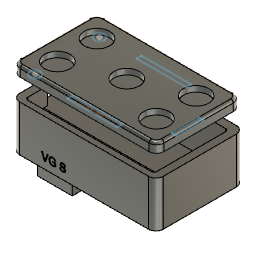
ESPBox and Lid (Autodesk Fusion 360 design; units mm, degrees)
Autodesk Fusion 360 part; units mm, degrees
sketch "Skizze1" plane through (0, 0, 0) normal (0, 0, 1) x (1, 0, 0) in component "Box1"
  line L0 (29, 17.25) -> (-29, 17.25)
  line L1 (-29, 17.25) -> (-29, -17.25)
  line L2 (-29, -17.25) -> (29, -17.25)
  line L3 (29, -17.25) -> (29, 17.25)
  line L4 (29, 17.25) -> (-29, -17.25) construction
  line L5 (-29, 17.25) -> (29, -17.25) construction
  dimension "d1" = 58
  dimension "d2" = 34.5
  constraint horizontal L0
  constraint perpendicular L0 L1
  constraint parallel L0 L2
  constraint parallel L1 L3
  constraint coincident L4 origin
  constraint coincident L5 origin
  measures "d1" distance of L1.end L2.end
  measures "d2" distance of L0.end L1.end
extrude "Extrusion1" add sketch "Skizze1" along normal blind 18.5 makes body 1 in component "Box1"
sketch "Skizze2" plane through (0, 0, 18.5) normal (0, 0, 1) x (-1, 0, 0) in component "Box1"
  line L0 (-29, 17.25) -> (-29, -17.25)
  line L1 (-29, -17.25) -> (29, -17.25)
  line L2 (29, -17.25) -> (29, 17.25)
  line L3 (29, 17.25) -> (-29, 17.25)
  line L4 (-26, -15) -> (26, -15)
  line L5 (26, -15) -> (26, 15)
  line L6 (26, 15) -> (-26, 15)
  line L7 (-26, 15) -> (-26, -15)
  line L8 (-26, -15) -> (26, 15) construction
  line L9 (26, -15) -> (-26, 15) construction
  dimension "d5" = 52
  dimension "d6" = 30
  constraint horizontal L4
  constraint perpendicular L4 L5
  constraint parallel L4 L6
  constraint parallel L5 L7
  constraint coincident L8 origin
  constraint coincident L9 origin
  measures "d5" distance of L5.end L6.end
  measures "d6" distance of L4.end L5.end
extrude "Extrusion2" cut sketch "Skizze2" against normal up to surface (15.5 mm away) contours L4 L5 L6 L7 bodies 1 in component "Box1"
fillet "Abrundung1" radius 1 4 edges at (26, 15, 10.75) (-26, 15, 10.75) (-26, -15, 10.75) (26, -15, 10.75) on bodies 1 in component "Box1"
fillet "Abrundung2" radius 3 4 edges at (29, -17.25, 9.25) (-29, -17.25, 9.25) (-29, 17.25, 9.25) (29, 17.25, 9.25) on bodies 1 in component "Box1"
sketch "Skizze3" plane through (0, 0, 3) normal (0, 0, 1) x (-1, 0, 0) in component "Box1"
  arc A0 (-25, 15) -> (-26, 14) centre (-25, 14) ccw
  line L0 (-26, 14) -> (-26, -14)
  arc A1 (-26, -14) -> (-25, -15) centre (-25, -14) ccw
  line L1 (-25, -15) -> (25, -15)
  arc A2 (25, -15) -> (26, -14) centre (25, -14) ccw
  line L2 (26, -14) -> (26, 14)
  arc A3 (26, 14) -> (25, 15) centre (25, 14) ccw
  line L3 (25, 15) -> (-25, 15)
  line L4 (17, 12.0213) -> (17, 15.0213)
  line L5 (17, 15.0213) -> (7, 15.0213)
  line L6 (7, 15.0213) -> (7, 12.0213)
  line L7 (7, 12.0213) -> (17, 12.0213)
  line L8 (17, 12.0213) -> (17, 15.0213)
  dimension "d15" = 10
  dimension "d16" = 3
  constraint vertical L4
  constraint horizontal L5
  constraint vertical L6
  constraint horizontal L7
  constraint vertical L8
  measures "d15" distance of L4.end L5.end
  measures "d16" distance of L4.end L4.start
extrude "Extrusion3" cut sketch "Skizze3" against normal blind 4 contours L3 L4 L6 L7 L8 bodies 1 in component "Box1"
sketch "Skizze4" plane through (0, 0, 3) normal (0, 0, 1) x (-1, 0, 0) in component "Box1"
  line L0 (17, 15) -> (17, 12.0213)
  line L1 (17, 12.0213) -> (7, 12.0213)
  line L2 (7, 12.0213) -> (7, 15)
  line L3 (7, 15) -> (-25, 15)
  arc A0 (-25, 15) -> (-26, 14) centre (-25, 14) ccw
  line L4 (-26, 14) -> (-26, -14)
  arc A1 (-26, -14) -> (-25, -15) centre (-25, -14) ccw
  line L5 (-25, -15) -> (25, -15)
  arc A2 (25, -15) -> (26, -14) centre (25, -14) ccw
  line L6 (26, -14) -> (26, 14)
  arc A3 (26, 14) -> (25, 15) centre (25, 14) ccw
  line L7 (25, 15) -> (17, 15)
  line L8 (-26, -7.5) -> (26, -7.5)
  line L9 (26, -7.5) -> (26, 7.5)
  line L10 (26, 7.5) -> (-26, 7.5)
  line L11 (-26, 7.5) -> (-26, -7.5)
  line L12 (-26, -7.5) -> (26, 7.5) construction
  line L13 (26, -7.5) -> (-26, 7.5) construction
  dimension "d19" = 52
  dimension "d20" = 15
  constraint horizontal L8
  constraint perpendicular L8 L9
  constraint parallel L8 L10
  constraint parallel L9 L11
  constraint coincident L12 origin
  constraint coincident L13 origin
  measures "d19" distance of L9.end L10.end
  measures "d20" distance of L8.end L9.end
extrude "Extrusion4" add sketch "Skizze4" along normal blind 8.5 contours L4 L6 L8 L9 L10 L11 bodies 1 in component "Box1"
sketch "Skizze5" plane through (-26, 0, 0) normal (1, 0, 0) x (0, 1, 0) in component "Box1"
  line L0 (7.5, 11.5) -> (7.5, 3)
  line L1 (7.5, 3) -> (14, 3)
  line L2 (14, 3) -> (14, 18.5)
  line L3 (14, 18.5) -> (-14, 18.5)
  line L4 (-14, 18.5) -> (-14, 3)
  line L5 (-14, 3) -> (-7.5, 3)
  line L6 (-7.5, 3) -> (-7.5, 11.5)
  line L7 (-7.5, 11.5) -> (7.5, 11.5)
  line L8 (5, 18.5) -> (-5, 18.5)
  line L9 (-5, 18.5) -> (-5, 11.5)
  line L10 (-5, 11.5) -> (5, 11.5)
  line L11 (5, 11.5) -> (5, 18.5)
  line L12 (5, 18.5) -> (-5, 11.5) construction
  line L13 (-5, 18.5) -> (5, 11.5) construction
  point P0 (0, 15)
  dimension "d23" = 10
  dimension "d24" = 7
  constraint horizontal L8
  constraint perpendicular L8 L9
  constraint parallel L8 L10
  constraint parallel L9 L11
  constraint coincident L12 P0
  constraint coincident L13 P0
  measures "d23" distance of L9.end L10.end
  measures "d24" distance of L8.end L9.end
extrude "Extrusion5" cut sketch "Skizze5" against normal blind 3 contours L3 L7 L8 L9 L10 L11 bodies 1 in component "Box1"
move_face "Flächen versetzen3" offset -0.5 3 faces at (-17, -13.0142, 2) (-10.3333, -12.0213, 2) (-7, -14.0071, 2) on bodies 1 in component "Box1"
sketch "Skizze2 (2)" plane through (0, -16.4091, 0) normal (0, -1, 0) x (1, 0, 0)
  line L0 (24.1814, 0.2273) -> (24.1814, 18.7273)
  line L1 (-27.8186, 18.7273) -> (-27.8186, 0.2273)
  line L2 (-19, 1.7273) -> (-5.8886, 1.7273) construction
  line L3 (-5.8886, 1.7273) -> (-5.8886, 6) construction
  line L4 (-5.8886, 6) -> (-19, 6) construction
  line L5 (-19, 6) -> (-19, 1.7273) construction
  line L6 (-27.8186, 0.2273) -> (24.1814, 0.2273)
  line L7 (24.1814, 18.7273) -> (-27.8186, 18.7273)
  dimension "d47" = 3
  text T0 "VG S" font "Arial" height 3 align left top in box 13.1114 x 4.2727 at (-19, 1.7273) x (1, 0) y (0, 1) spacing 1 kerned
extrude "Extrusion8" cut sketch "Skizze2 (2)" against normal blind 0.5 text T0 sketch seen with x (1, 0, 0) y (0, 1, 0) z (0, 0, 1) at (1.8186, -0.8409, -0.2273) bodies 1 in component "Box1"
move_face "Flächen versetzen5" offset 1 1 faces at (8.6667, 17.25, 6.1667) on bodies 1 in component "Box1"
move_face "Flächen versetzen6" offset -1 2 faces at (-28, 5, 16.1667) (-27, -5, 16.1667) on bodies 1 in component "Box1"
ref_plane "Arbeitsebene1" through (0, 0, 17) normal (0, 0, 1) x (1, 0, 0) in component "Deckel"
sketch "Skizze2 (3)" plane through (0, 0, 17) normal (0, 0, 1) x (1, 0, 0) in component "Deckel"
  line L0 (29, 17) -> (-29, 17)
  line L1 (-29, 17) -> (-29, -17)
  line L2 (-29, -17) -> (29, -17)
  line L3 (29, -17) -> (29, 17)
  line L4 (29, 17) -> (-29, -17) construction
  line L5 (-29, 17) -> (29, -17) construction
  constraint horizontal L0
  constraint perpendicular L0 L1
  constraint parallel L0 L2
  constraint parallel L1 L3
  constraint coincident L4 origin
  constraint coincident L5 origin
extrude "Extrusion1'" add sketch "Skizze2 (3)" along normal blind 4 separate body makes body 2 in component "Deckel"
fillet "Abrundung1'" radius 3 4 edges at (29, -17, 19) (29, 17, 19) (-29, 17, 19) (-29, -17, 19) on bodies 2 in component "Deckel"
fillet "Abrundung2'" radius 1 8 edges at (28.1213, -16.1213, 21) (29, 0, 21) (28.1213, 16.1213, 21) (0, 17, 21) (-28.1213, 16.1213, 21) (-29, 0, 21) (-28.1213, -16.1213, 21) (0, -17, 21) on bodies 2 in component "Deckel"
sketch "Skizze4 (2)" plane through (0, 0, 17) normal (0, 0, -1) x (1, 0, 0) in component "Deckel"
  arc A0 (-26, 17) -> (-29, 14) centre (-26, 14) ccw
  line L0 (-29, 14) -> (-29, -14)
  arc A1 (-29, -14) -> (-26, -17) centre (-26, -14) ccw
  line L1 (-26, -17) -> (26, -17)
  arc A2 (26, -17) -> (29, -14) centre (26, -14) ccw
  line L2 (29, -14) -> (29, 14)
  arc A3 (29, 14) -> (26, 17) centre (26, 14) ccw
  line L3 (26, 17) -> (-26, 17)
  line L4 (-9, -15) -> (11, -15)
  line L5 (11, -15) -> (11, -13)
  line L6 (11, -13) -> (-9, -13)
  line L7 (-9, -13) -> (-9, -15)
  line L8 (26, 6) -> (24, 6)
  line L9 (24, 6) -> (24, -5)
  line L10 (24, -5) -> (26, -5)
  line L11 (26, -5) -> (26, 6)
  circle A4 centre (-24, -13) radius 2
  circle A5 centre (-24, 13) radius 2
  line L12 (11, 15) -> (-9, 15)
  line L13 (-9, 15) -> (-9, 13)
  line L14 (-9, 13) -> (11, 13)
  line L15 (11, 13) -> (11, 15)
  line L16 (11, 15) -> (-9, 13) construction
  line L17 (-9, 15) -> (11, 13) construction
  point P0 (1, 14)
  dimension "d62" = 4
  dimension "d86" = 4
  constraint horizontal L4
  constraint vertical L5
  constraint horizontal L6
  constraint vertical L7
  constraint horizontal L8
  constraint vertical L9
  constraint horizontal L10
  constraint vertical L11
  constraint horizontal L12
  constraint perpendicular L12 L13
  constraint parallel L12 L14
  constraint parallel L13 L15
  constraint coincident L16 P0
  constraint coincident L17 P0
  measures "d62" diameter of A4
  measures "d86" diameter of A5
extrude "Extrusion9" add sketch "Skizze4 (2)" along normal blind 1 contours L12 L13 L14 L15 bodies 2 in component "Deckel"
extrude "Extrusion8'" add sketch "Skizze4 (2)" along normal blind 2 contours A4 | A5 bodies 2 in component "Deckel"
extrude "Extrusion3'" add sketch "Skizze4 (2)" along normal blind 1 contours L4 L5 L6 L7 | L8 L9 L10 L11 bodies 2 in component "Deckel"
sketch "Skizze7" plane through (0, -11.5213, 0) normal (0, -1, 0) x (1, 0, 0) in component "Box1"
  line L0 (-17.5, 0) -> (-6.5, 0)
  line L1 (-6.5, 0) -> (-6.5, 3)
  line L2 (-6.5, 3) -> (-17.5, 3)
  line L3 (-17.5, 3) -> (-17.5, 0)
  line L4 (-11.5, 0) -> (-9.5, 0)
  line L5 (-9.5, 0) -> (-9.5, 3)
  line L6 (-9.5, 3) -> (-11.5, 3)
  line L7 (-11.5, 3) -> (-11.5, 0)
  dimension "d71" = 2
  dimension "d72" = 3
  constraint horizontal L4
  constraint vertical L5
  constraint horizontal L6
  constraint vertical L7
  constraint coincident L0 L4.start
  measures "d71" distance of L4.start L4.end
  measures "d72" distance of L4.start L6.end
extrude "Extrusion9'" add sketch "Skizze7" along normal up to surface (3.4787 mm away) contours L0 L2 L4 L5 L6 L7 bodies 1 in component "Box1"
sketch "Skizze3 (2)" plane through (0, 0, 21) normal (0, 0, 1) x (-1, 0, 0)
  arc A0 (-26, 16) -> (-28, 14) centre (-26, 14) ccw
  line L0 (-28, 14) -> (-28, -14)
  arc A1 (-28, -14) -> (-26, -16) centre (-26, -14) ccw
  line L1 (-26, -16) -> (26, -16)
  arc A2 (26, -16) -> (28, -14) centre (26, -14) ccw
  line L2 (28, -14) -> (28, 14)
  arc A3 (28, 14) -> (26, 16) centre (26, 14) ccw
  line L3 (26, 16) -> (-26, 16)
  circle A4 centre (-20, 8) radius 5.1
  circle A5 centre (20, 8) radius 5.1
  circle A6 centre (20, -8) radius 5.1
  circle A7 centre (-20, -8) radius 5.1
  circle A8 centre (0, 0) radius 5.1
  dimension "d75" = 10.2
  dimension "d76" = 10.2
  dimension "d77" = 10.2
  dimension "d78" = 10.2
  dimension "d79" = 10.2
  constraint coincident A8.centre origin
  measures "d75" diameter of A4
  measures "d76" diameter of A5
  measures "d77" diameter of A6
  measures "d78" diameter of A7
  measures "d79" diameter of A8
extrude "Extrusion6" cut sketch "Skizze3 (2)" against normal blind 2.3 contours A4 | A5 | A6 | A7 | A8 bodies 2 in component "Deckel"
sketch "Skizze4 (3)" plane through (0, 0, 17) normal (0, 0, -1) x (1, 0, 0)
  line L0 (-9, -13) -> (11, -13)
  line L1 (11, -13) -> (11, -15)
  line L2 (11, -15) -> (-9, -15)
  line L3 (-9, -15) -> (-9, -13)
  line L4 (26, -5) -> (24, -5)
  line L5 (24, -5) -> (24, 6)
  line L6 (24, 6) -> (26, 6)
  line L7 (26, 6) -> (26, -5)
  arc A0 (-26, 17) -> (-29, 14) centre (-26, 14) ccw
  line L8 (-29, 14) -> (-29, -14)
  arc A1 (-29, -14) -> (-26, -17) centre (-26, -14) ccw
  line L9 (-26, -17) -> (26, -17)
  arc A2 (26, -17) -> (29, -14) centre (26, -14) ccw
  line L10 (29, -14) -> (29, 14)
  arc A3 (29, 14) -> (26, 17) centre (26, 14) ccw
  line L11 (26, 17) -> (-26, 17)
  line L12 (-19, 9) -> (-2, 9)
  line L13 (-2, 9) -> (-2, -8)
  line L14 (-2, -8) -> (-19, -8)
  line L15 (-19, -8) -> (-19, 9)
  circle A4 centre (-24, 13) radius 2
  circle A5 centre (-24, -13) radius 2
  line L16 (11, 13) -> (-9, 13)
  line L17 (-9, 13) -> (-9, 15)
  line L18 (-9, 15) -> (11, 15)
  line L19 (11, 15) -> (11, 13)
  constraint horizontal L12
  constraint vertical L13
  constraint horizontal L14
  constraint vertical L15
extrude "Extrusion7" add sketch "Skizze4 (3)" along normal blind 4 contours L12 L13 L14 L15 bodies 2 in component "Deckel"
sketch "Skizze5 (2)" plane through (0, 0, 0) normal (0, 0, -1) x (1, 0, 0)
  line L0 (-11.5, 11.5213) -> (-17.5, 11.5213)
  line L1 (-17.5, 11.5213) -> (-17.5, 15)
  line L2 (-17.5, 15) -> (-11.5, 15)
  line L3 (-11.5, 15) -> (-11.5, 11.5213)
  arc A0 (-29, -15.25) -> (-26, -18.25) centre (-26, -15.25) ccw
  line L4 (-26, -18.25) -> (26, -18.25)
  arc A1 (26, -18.25) -> (29, -15.25) centre (26, -15.25) ccw
  line L5 (29, -15.25) -> (29, 14.25)
  arc A2 (29, 14.25) -> (26, 17.25) centre (26, 14.25) ccw
  line L6 (26, 17.25) -> (-26, 17.25)
  arc A3 (-26, 17.25) -> (-29, 14.25) centre (-26, 14.25) ccw
  line L7 (-29, 14.25) -> (-29, -15.25)
  line L8 (-9.5, 11.5213) -> (-9.5, 15)
  line L9 (-9.5, 15) -> (-6.5, 15)
  line L10 (-6.5, 15) -> (-6.5, 11.5213)
  line L11 (-6.5, 11.5213) -> (-9.5, 11.5213)
  line L12 (-10, 17) -> (-19, 17)
  line L13 (-19, 17) -> (-19, 9.5213)
  line L14 (-19, 9.5213) -> (-10, 9.5213)
  line L15 (-10, 9.5213) -> (-10, 17)
  line L16 (-10, 17) -> (-19, 9.5213) construction
  line L17 (-19, 17) -> (-10, 9.5213) construction
  line L18 (-11.5, 15) -> (-17.5, 15)
  line L19 (-17.5, 15) -> (-17.5, 11.5213)
  line L20 (-17.5, 11.5213) -> (-11.5, 11.5213)
  line L21 (-11.5, 11.5213) -> (-11.5, 15)
  line L22 (-11.5, 15) -> (-17.5, 11.5213) construction
  line L23 (-17.5, 15) -> (-11.5, 11.5213) construction
  line L24 (-6.5, 15) -> (-9.5, 15)
  line L25 (-9.5, 15) -> (-9.5, 11.5213)
  line L26 (-9.5, 11.5213) -> (-6.5, 11.5213)
  line L27 (-6.5, 11.5213) -> (-6.5, 15)
  line L28 (-6.5, 15) -> (-9.5, 11.5213) construction
  line L29 (-9.5, 15) -> (-6.5, 11.5213) construction
  line L30 (-5, 17) -> (-11, 17)
  line L31 (-11, 17) -> (-11, 9.5213)
  line L32 (-11, 9.5213) -> (-5, 9.5213)
  line L33 (-5, 9.5213) -> (-5, 17)
  line L34 (-5, 17) -> (-11, 9.5213) construction
  line L35 (-11, 17) -> (-5, 9.5213) construction
  point P0 (-14.5, 13.2607)
  point P1 (-14.5, 13.2607)
  point P2 (-8, 13.2607)
  point P3 (-8, 13.2607)
  constraint horizontal L12
  constraint perpendicular L12 L13
  constraint parallel L12 L14
  constraint parallel L13 L15
  constraint coincident L16 P1
  constraint coincident L17 P1
  constraint horizontal L18
  constraint perpendicular L18 L19
  constraint parallel L18 L20
  constraint parallel L19 L21
  constraint coincident L2.end L3.start
  constraint coincident L22 P1
  constraint coincident L23 P1
  constraint coincident P1 P0
  constraint horizontal L24
  constraint perpendicular L24 L25
  constraint parallel L24 L26
  constraint parallel L25 L27
  constraint coincident L9.end L10.start
  constraint coincident L28 P3
  constraint coincident L29 P3
  constraint horizontal L30
  constraint perpendicular L30 L31
  constraint parallel L30 L32
  constraint parallel L31 L33
  constraint coincident L34 P3
  constraint coincident L35 P3
  constraint coincident P3 P2
extrude "Extrusion10" add sketch "Skizze5 (2)" along normal blind 4 contours L12 L14 L15 L30 L31 L32 | L15 L30 L32 L33 | L12 L13 L14 L31 bodies 1 in component "Box1"
component "Box1" placed x (1, 0, 0) y (0, 1, 0) z (0, 0, 1) at (0, 0, 0)
component "Deckel" placed x (1, 0, 0) y (0, 1, 0) z (0, 0, 1) at (0, 0, 10)
